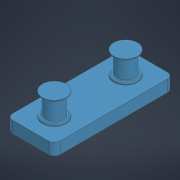
# Autodesk Inventor part: Soporte Engrane
Saved by Autodesk Inventor 2022 (Build 260153000, 153)
## iProperties
Created: 2022-05-04
Part Number: Soporte Engrane
Material: Genérico
Document SubType Name: Modeling
Designer: aleon
Density: 1 g/cm^3
Appearance: Valor por defecto
Author: aleon
Autodesk Inventor part; units mm, degrees
ref_plane "YZ Plane" through (0, 0, 0) normal (1, 0, 0) x (0, 1, 0)
ref_plane "XZ Plane" through (0, 0, 0) normal (0, 1, 0) x (-1, 0, 0)
ref_plane "XY Plane" through (0, 0, 0) normal (0, 0, 1) x (1, 0, 0)
sketch "Boceto1" plane through (0, 0, 0) normal (0, 1, 0) x (-1, 0, 0)
  line L0 (-15, -50) -> (15, -50)
  line L1 (20, -45) -> (20, 45)
  line L2 (15, 50) -> (-15, 50)
  line L3 (-20, 45) -> (-20, -45)
  arc A0 (-15, 50) -> (-20, 45) centre (-15, 45) ccw
  arc A1 (-20, -45) -> (-15, -50) centre (-15, -45) ccw
  arc A2 (15, -50) -> (20, -45) centre (15, -45) ccw
  arc A3 (20, 45) -> (15, 50) centre (15, 45) ccw
  circle A4 centre (0, 28.75) radius 10
  circle A5 centre (0.1077, -28.75) radius 10
  point P0 (0, 0)
  dimension "d3" = 5
  dimension "d4" = 5
  dimension "d5" = 5
  dimension "d6" = 5
  dimension "d7" = 20
  dimension "d8" = 20
  dimension "d10" = 28.75
  dimension "d11" = 28.75
  constraints: 8 end point, 8 point on circle, 8 tangent, 6 centre point, 2 parallel, 1 horizontal, 1 perpendicular, 1 vertical alignment
  measures "d3" radius of A0
  measures "d4" radius of A1
  measures "d5" radius of A2
  measures "d6" radius of A3
  measures "d7" diameter of A4
  measures "d8" diameter of A5
  measures "d10" distance of point (0, 0) A4.centre
  measures "d11" vertical distance of point (0, 0) A5.centre
extrude "Extrusión1" add sketch "Boceto1" along normal blind 10
extrude "Extrusión2" add sketch "Boceto1" along normal blind 12 contours A4 | A5
sketch "Boceto2" plane through (0, 12, 28.75) normal (0, 1, 0) x (1, 0, 0)
  circle A0 centre (0, 0) radius 7.5
  circle A1 centre (-0.1077, 57.5) radius 7.5
  circle A2 centre (-0.1077, 57.5) radius 10 projected
  circle A3 centre (0, 0) radius 10 projected
  point P0 (0, 28.75)
  dimension "d16" = 15
  dimension "d17" = 15
  dimension "d26" = 2.5
  constraints: 2 centre point, 2 coincident
  measures "d16" diameter of A0
  measures "d17" diameter of A1
  measures "d26" radial gap between concentric circles of A3 A0
extrude "Extrusión3" add sketch "Boceto2" along normal blind 15 contours A0 | A1
sketch "Boceto3" plane through (0, 27, 28.75) normal (0, 1, 0) x (1, 0, 0)
  circle A0 centre (0, 0) radius 7.5 projected
  circle A1 centre (0, 0) radius 10
  circle A2 centre (-0.1077, 57.5) radius 10
  circle A3 centre (-0.1077, 57.5) radius 10 projected
  point P0 (0, 28.75)
  dimension "d20" = 20
  dimension "d21" = 20
  constraints: 3 coincident, 2 centre point
  measures "d20" diameter of A1
  measures "d21" diameter of A2
extrude "Extrusión4" add sketch "Boceto3" along normal blind 2 contours A0 | A1 | A2
fillet "Empalme1" radius 1.5 4 edges at (10, 12, 28.75) (-10, 27, 28.75) (9.8923, 12, -28.75) (-10.1077, 27, -28.75)
